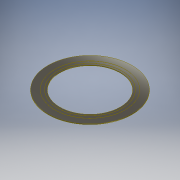
# Autodesk Inventor part: Gasket
Saved by Autodesk Inventor 2016 (Build 200138000, 138)
## iProperties
Created: 2018-11-05
Part Number: Gasket
Material: Steel, Carbon
Document SubType Name: Modeling
Designer: Wijaya
Mass: 2529.27 g
Surface Area: 1906.84 cm^2
Volume: 322.2 cm^3
Density: 7.85 g/cm^3
Appearance: Silver
Author: Wijaya
Autodesk Inventor part; units mm, degrees
ref_plane "YZ Plane" through (0, 0, 0) normal (1, 0, 0) x (0, 1, 0)
ref_plane "XZ Plane" through (0, 0, 0) normal (0, 1, 0) x (-1, 0, 0)
ref_plane "XY Plane" through (0, 0, 0) normal (0, 0, 1) x (1, 0, 0)
sketch "Sketch1" plane through (0, 0, 0) normal (0, 0, 1) x (1, 0, 0)
  circle A0 centre (0, 0) radius 174.65
  circle A1 centre (0, 0) radius 242.95
  circle A2 centre (0, 0) radius 185.8
  circle A3 centre (0, 0) radius 203.2
  dimension "d0" = 349.3
  dimension "d1" = 485.9
  dimension "d2" = 371.6
  dimension "d3" = 406.4
  constraints: 4 centre point, 4 coincident
  measures "d0" diameter of A0
  measures "d1" diameter of A1
  measures "d2" diameter of A2
  measures "d3" diameter of A3
extrude "Extrusion1" add sketch "Sketch1" along normal mid plane 3.33
extrude "Extrusion2" add sketch "Sketch1" along normal mid plane 4.45 contours A3
body "Solid1"
